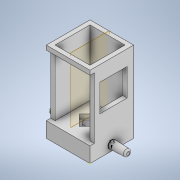
# Autodesk Inventor part: latticeChamberv6b
Saved by Autodesk Inventor 2020.5 (Build 245400000, 400)
## iProperties
Created: 2022-09-01
Part Number: latticeChamberv6b
Material: Generic
Document SubType Name: Modeling
Designer: ISS
Density: 1 g/cm^3
Appearance: Default
Author: ISS
Autodesk Inventor part; units mm, degrees
ref_plane "YZ Plane" through (0, 0, 0) normal (1, 0, 0) x (0, 1, 0)
sketch "Sketch1" plane through (0, 0, 0) normal (0, 1, 0) x (-1, 0, 0)
  line L0 (0, 0) -> (20, 0)
  line L1 (20, 0) -> (20, -20)
  line L2 (20, -20) -> (0, -20)
  line L3 (0, -20) -> (0, 0)
  dimension "d0" = 20
  dimension "d1" = 20
  constraints: 8 end point, 2 parallel, 1 horizontal, 1 perpendicular
  measures "d0" distance of L1.end L2.end
  measures "d1" distance of L0.end L1.end
extrude "Extrusion1" add sketch "Sketch1" along normal blind 10
sketch "Sketch4" plane through (0, 10, 0) normal (0, 1, 0) x (1, 0, 0)
  line L0 (0, 20) -> (-20, 20) projected
  line L1 (-20, 20) -> (-20, 0) projected
  line L2 (-20, 0) -> (0, 0) projected
  line L3 (0, 0) -> (0, 20) projected
  line L4 (0, 20) -> (-20, 20) projected
  line L5 (-20, 20) -> (0, 0)
  line L6 (-10.1768, 10.1768) -> (-7.7019, 12.6517)
  line L7 (-7.7019, 12.6517) -> (-5.227, 10.1768)
  line L8 (-5.227, 10.1768) -> (-7.7019, 7.7019)
  line L9 (-7.7019, 7.7019) -> (-10.1768, 10.1768)
  line L10 (-10.1768, 10.1768) -> (-12.6517, 7.7019)
  line L11 (-12.6517, 7.7019) -> (-15.1265, 10.1768)
  line L12 (-15.1265, 10.1768) -> (-12.6517, 12.6517)
  line L13 (-12.6517, 12.6517) -> (-10.1768, 10.1768)
  line L14 (-12.6517, 12.6517) -> (-10.1768, 15.1265)
  line L15 (-10.1768, 15.1265) -> (-7.7019, 12.6517)
  line L16 (-7.7019, 12.6517) -> (-10.1768, 10.1768)
  line L17 (-10.1768, 10.1768) -> (-12.6517, 12.6517)
  line L18 (-12.6517, 7.7019) -> (-10.1768, 10.1768)
  line L19 (-10.1768, 10.1768) -> (-7.7019, 7.7019)
  line L20 (-7.7019, 7.7019) -> (-10.1768, 5.227)
  line L21 (-10.1768, 5.227) -> (-12.6517, 7.7019)
  dimension "d10" = 3.5
  dimension "d11" = 3.5
  dimension "d12" = 3.5
  dimension "d13" = 3.5
  constraints: 34 end point, 8 parallel, 4 perpendicular
  measures "d10" distance of L7.end L8.end
  measures "d11" distance of L6.end L7.end
  measures "d12" distance of L11.end L12.end
  measures "d13" distance of L10.end L11.end
extrude "Extrusion3" cut sketch "Sketch4" against normal blind 8 contours L14 L15 L6 L5 | L5 L10 L11 L12 | L20 L21 L10 L5 | L5 L6 L7 L8
sketch "Sketch5" plane through (0, 10, 0) normal (0, 1, 0) x (1, 0, 0)
  line L0 (-5.227, 10.1768) -> (-10.1768, 5.227) projected
  line L1 (-10.1768, 5.227) -> (-15.1265, 10.1768) projected
  line L2 (-15.1265, 10.1768) -> (-10.1768, 15.1265) projected
  line L3 (-10.1768, 15.1265) -> (-5.227, 10.1768) projected
  line L4 (0, 20) -> (-20, 20) projected
  line L5 (-20, 20) -> (-20, 0) projected
  line L6 (-20, 0) -> (0, 0) projected
  line L7 (0, 0) -> (0, 20) projected
  line L8 (-18, 18) -> (-2, 18)
  line L9 (-2, 18) -> (-2, 2)
  line L10 (-2, 2) -> (-18, 2)
  line L11 (-18, 2) -> (-18, 18)
  line L12 (-18, 2) -> (-18, 0)
  line L13 (-2, 2) -> (-2, 0)
  line L14 (-20, 0) -> (0, 0) projected
  line L15 (-18, 2) -> (-20, 2)
  line L16 (-20, 20) -> (-20, 0) projected
  line L17 (-2, 2) -> (0, 2)
  line L18 (0, 0) -> (0, 20) projected
  point P0 (0, 2)
  dimension "d16" = 2
  constraints: 16 end point, 5 point on line, 3 perpendicular, 3 other
  measures "d16" distance between parallel lines of L4 L8
extrude "Extrusion4" add sketch "Sketch5" along normal blind 27 contours L7 L17 L9 L8 L11 L15 L5 L4
ref_plane "Work Plane1" through (-10, 10, -2) normal (1, 0, 0) x (0, 0, -1)
sketch "Sketch6" plane through (-10, 10, -2) normal (1, 0, 0) x (0, 0, -1)
  line L0 (3.227, 0) -> (8.1768, 0) projected
  line L1 (3.227, 0) -> (3.227, -8) projected
  line L2 (3.227, -8) -> (8.1768, -8) projected
  line L3 (8.1768, 0) -> (8.1768, -8) projected
  line L4 (8.1768, 0) -> (13.1265, 0) projected
  line L5 (8.1768, 0) -> (8.1768, -8) projected
  line L6 (8.1768, -8) -> (13.1265, -8) projected
  line L7 (13.1265, 0) -> (13.1265, -8) projected
  line L8 (16, 0) -> (0, 0) projected
  line L9 (16, 0) -> (16, 27) projected
  line L10 (0, 27) -> (16, 27) projected
  line L11 (0, 0) -> (0, 27) projected
  line L12 (8.1768, 0) -> (8.1768, -8) projected
  line L13 (8.1768, -8) -> (8.1768, -7.25)
  circle A0 centre (8.1768, -7.25) radius 0.75
  point P0 (-2, -10)
  dimension "d20" = 0.75
  dimension "d21" = 1.5
  constraints: 2 end point, 1 centre point, 1 coincident, 1 point on line
  measures "d20" distance of L2.end L13.end
  measures "d21" diameter of A0
extrude "Extrusion5" cut sketch "Sketch6" along normal mid plane 27 contours A0 L3 | L3 A0
ref_plane "Work Plane2" through (-20, 0, -10) normal (0, 0, 1) x (1, 0, 0)
sketch "Sketch7" plane through (-20, 0, -10) normal (0, 0, 1) x (1, 0, 0)
  line L0 (20, 0) -> (0, 0) projected
  line L1 (0, 0) -> (0, 37) projected
  line L2 (20, 37) -> (0, 37) projected
  line L3 (20, 0) -> (20, 37) projected
  arc A0 (14.773, 3.5) -> (14.773, 2) centre (14.773, 2.75) ccw projected
  arc A1 (14.773, 3.5) -> (14.773, 2) centre (14.773, 2.75) ccw projected
  line L4 (20, 3.5) -> (20, 2) projected
  line L5 (20, 3.5) -> (27.5, 3.5)
  line L6 (27.5, 3.5) -> (27.5, 2)
  line L7 (27.5, 2) -> (20, 2)
  line L8 (20, 2) -> (20, 3.5)
  line L9 (20, 3.5) -> (20, 4.5)
  line L10 (20, 0) -> (20, 37) projected
  line L11 (27.5, 3.5) -> (27.5, 3.5246)
  line L12 (26.775, 4.2742) -> (20, 4.5)
  arc A2 (27.5, 3.5246) -> (26.775, 4.2742) centre (26.75, 3.5246) ccw
  line L13 (20, 3.5) -> (20, 2) projected
  line L14 (20, 2.75) -> (27.5, 2.75)
  point P0 (27.5, 4.25)
  dimension "d25" = 7.5
  dimension "d26" = 1
  dimension "d27" = 0.75
  dimension "d28" = 0.75
  constraints: 16 end point, 3 point on line, 2 midpoint, 2 parallel, 2 point on circle, 2 tangent, 1 centre point, 1 horizontal, 1 perpendicular, 1 vertical
  measures "d25" distance of L6.end L7.end
  measures "d26" distance of L4.start L9.end
  measures "d27" distance of L5.end point (27.5, 4.25)
  measures "d28" radius of A2
revolve "Revolution1" add sketch "Sketch7" angle 360 about axis through (0, 2.75, -10) along (1, 0, 0) contours L3 L12 A2 L11 L5
mirror "Mirror1" about plane through (-10, 10, -2) normal (1, 0, 0) of "Revolution1"
sketch "Sketch8" plane through (-20, 10, -2) normal (0, 0, 1) x (1, 0, 0)
  line L0 (2, 0) -> (0, 0) projected
  line L1 (2, 0) -> (2, 27) projected
  line L2 (0, 27) -> (2, 27) projected
  line L3 (0, 0) -> (0, 27) projected
  line L4 (20, 0) -> (18, 0) projected
  line L5 (20, 0) -> (20, 27) projected
  line L6 (18, 27) -> (20, 27) projected
  line L7 (18, 0) -> (18, 27) projected
  line L8 (20, 27) -> (0, 27) projected
  line L9 (0, 27) -> (20, 27)
  line L10 (20, 27) -> (20, 25)
  line L11 (20, 25) -> (0, 25)
  line L12 (0, 25) -> (0, 27)
  point P0 (20, -10)
  point P1 (0, 25)
  dimension "d30" = 20
  dimension "d31" = 2
  constraints: 8 end point, 2 parallel, 1 horizontal, 1 perpendicular
  measures "d30" distance of L10.end L11.end
  measures "d31" distance of L9.end L10.end
extrude "Extrusion6" add sketch "Sketch8" along normal blind 2 contours L11 L3 L2 L1 | L1 L8 L7 L11 | L7 L6 L5 L11
ref_plane "Work Plane3" through (0, 8, 0) normal (0, 1, 0) x (1, 0, 0)
sketch "Sketch9" plane through (0, 8, 0) normal (0, 1, 0) x (1, 0, 0)
  line L0 (-10.1768, 15.1265) -> (-5.227, 10.1768) projected
  line L1 (-15.1265, 10.1768) -> (-10.1768, 15.1265) projected
  line L2 (-10.1768, 5.227) -> (-15.1265, 10.1768) projected
  line L3 (-5.227, 10.1768) -> (-10.1768, 5.227) projected
  line L4 (-6.6412, 10.1768) -> (-10.1768, 13.7123)
  line L5 (-10.1768, 13.7123) -> (-13.7123, 10.1768)
  line L6 (-13.7123, 10.1768) -> (-10.1768, 6.6412)
  line L7 (-10.1768, 6.6412) -> (-6.6412, 10.1768)
  point P0 (0, 0)
  dimension "d35" = 1
  constraints: 8 end point, 3 other
  measures "d35" distance between parallel lines of L0 L4
extrude "Extrusion7" add sketch "Sketch9" against normal blind 6
extrude "Extrusion8" cut sketch "Sketch6" along normal mid plane 27 contours A0 L3 | L3 A0
sketch "Sketch10" plane through (0, 0, 0) normal (1, 0, 0) x (0, 0, -1)
  line L0 (0, 0) -> (20, 0) projected
  line L1 (20, 0) -> (20, 37) projected
  line L2 (20, 37) -> (0, 37) projected
  line L3 (0, 35) -> (0, 37) projected
  line L4 (2, 35) -> (0, 35) projected
  line L5 (2, 10) -> (2, 35) projected
  line L6 (0, 10) -> (2, 10) projected
  line L7 (0, 0) -> (0, 10) projected
  circle A0 centre (10, 2.75) radius 1.75 projected
  line L8 (2, 35) -> (10, 35)
  line L9 (10, 35) -> (4.5, 35)
  line L10 (4.5, 35) -> (4.5, 30)
  line L11 (4.5, 30) -> (17, 30)
  line L12 (17, 30) -> (17, 17.5)
  line L13 (17, 17.5) -> (4.5, 17.5)
  line L14 (4.5, 17.5) -> (4.5, 30)
  dimension "d40" = 5.5
  dimension "d41" = 5
  dimension "d42" = 12.5
  dimension "d43" = 12.5
  dimension "d44" = 8
  constraints: 14 end point, 2 horizontal, 2 parallel, 2 perpendicular, 1 point on line
  measures "d40" distance of L8.end L9.end
  measures "d41" distance of L9.end L10.end
  measures "d42" distance of L12.end L13.end
  measures "d43" distance of L11.end L12.end
  measures "d44" distance of L4.start L8.end
extrude "Extrusion9" cut sketch "Sketch10" against normal blind 6 contours L11 L12 L13 L14
move faces "Move1" translate (0, -3, 0) faces at (-8.5269, 8, -13.0052)
move faces "Move3" translate (0, -3, 0) faces at (-5.8013, 10, -5.8013)
sketch "Sketch12" plane through (-10, 10, -2) normal (1, 0, 0) x (0, 0, -1)
  circle A0 centre (8, -7.25) radius 0.75 projected
  point P0 (-2, -10)
extrude "Extrusion10" cut sketch "Sketch12" along normal mid plane 100
sketch "Sketch13" plane through (0, 0, 0) normal (1, 0, 0) x (0, 0, -1)
  arc A0 (10.0884, 3.4948) -> (10, 2) centre (10, 2.75) ccw projected
  circle A1 centre (10, 2.75) radius 1.75
  point P0 (0, 0)
  dimension "d58" = 3.5
  constraints: 1 centre point, 1 coincident
  measures "d58" diameter of A1
body "Solid1"
